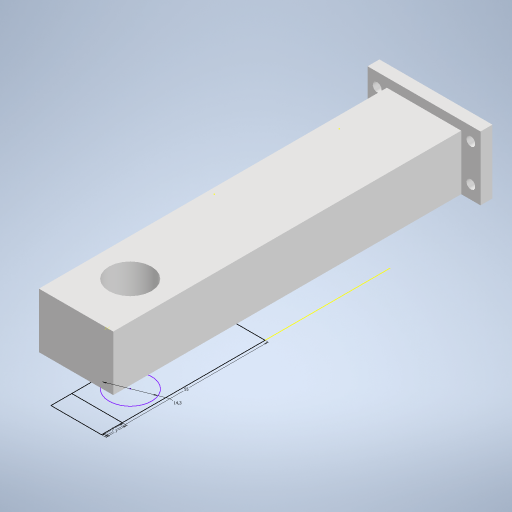
# Autodesk Inventor part: ramie_2
Saved by Autodesk Inventor 2023 (Build 270158000, 158)
## iProperties
Created: 2022-09-14
Part Number: ramie_2
Material: Generic
Document SubType Name: Modeling
Designer: Kamil
Density: 1 g/cm^3
Appearance: Default
Author: Kamil
Autodesk Inventor part; units mm, degrees
ref_plane "YZ Plane" through (0, 0, 0) normal (1, 0, 0) x (0, 1, 0)
ref_plane "XZ Plane" through (0, 0, 0) normal (0, 1, 0) x (-1, 0, 0)
ref_plane "XY Plane" through (0, 0, 0) normal (0, 0, 1) x (1, 0, 0)
sketch "Sketch14" plane through (0, 0, 0) normal (0, 0, 1) x (1, 0, 0)
  line L0 (0, 0) -> (17, 0)
  line L1 (17, 0) -> (17, 30)
  line L2 (17, 30) -> (0, 30)
  line L3 (0, 30) -> (0, 0)
  line L4 (-6, 36) -> (23, 36)
  line L5 (23, 36) -> (23, -6)
  line L6 (23, -6) -> (-6, -6)
  line L7 (-6, -6) -> (-6, 36)
  dimension "d55" = 17
  dimension "d56" = 30
  dimension "d57" = 6
  constraints: 16 end point, 4 parallel, 2 perpendicular, 1 horizontal, 3 other
  measures "d55" distance of L2.end L1.end
  measures "d56" distance of L1.end L0.end
  measures "d57" distance between parallel lines of L2 L4
extrude "Extrusion12" add sketch "Sketch14" against normal blind 3 contours L3 L2 L1 L0 | L4 L5 L6 L7
extrude "Extrusion13" add sketch "Sketch14" along normal blind 90 contours L3 L2 L1 L0
sketch "Sketch15" plane through (0, 0, 0) normal (0, -1, 0) x (1, 0, 0)
  line L0 (0, 0) -> (0, 90) projected
  line L1 (0, 90) -> (17.1111, 90)
  line L2 (0, 90) -> (17, 90)
  line L3 (17, 90) -> (17, 97)
  line L4 (17, 97) -> (0, 97)
  line L5 (0, 97) -> (0, 90)
  line L6 (17, 90) -> (0, 90) projected
  circle A0 centre (8.5, 78.8) radius 7.15
  line L7 (17, 0) -> (17, 90) projected
  line L8 (0, 97) -> (17, 97)
  line L9 (17, 97) -> (17, 42)
  line L10 (17, 42) -> (0, 42)
  line L11 (0, 42) -> (0, 97)
  dimension "d67" = 7
  dimension "d73" = 14.3
  dimension "d79" = 55
  constraints: 18 end point, 4 parallel, 3 horizontal, 2 perpendicular, 1 centre point, 1 point on line
  measures "d67" distance of L3.end L2.end
  measures "d73" diameter of A0
  measures "d79" distance of L8.end L9.end
extrude "Extrusion14" cut sketch "Sketch15" against normal blind 90 contours A0
extrude "Extrusion15" cut sketch "Sketch15" against normal blind 15.5 contours L0 L1 L7 L10
extrude "Extrusion17" add sketch "Sketch15" against normal blind 30 contours L5 L4 L3 L1
sketch "Sketch16" plane through (0, 0, 0) normal (0, -1, 0) x (1, 0, 0)
  line L0 (0, 0) -> (0, 97) projected
  line L1 (17, 0) -> (17, 97) projected
  line L2 (0, 97) -> (17, 97)
  line L3 (17, 97) -> (17, 90)
  line L4 (17, 90) -> (0, 90)
  line L5 (0, 90) -> (0, 97)
  dimension "d86" = 7
  constraints: 8 end point, 2 parallel, 1 horizontal, 1 perpendicular, 1 point on line
  measures "d86" distance of L2.end L3.end
extrude "Extrusion18" cut sketch "Sketch15" against normal blind 15.5 contours L5 L4 L3 L1
sketch "Sketch21" plane through (0, 15.5, 97) normal (0, 0, 1) x (1, 0, 0)
  line L0 (0, 14.5) -> (17, 14.5) projected
  line L1 (0, 14.5) -> (0, 16.5)
  line L2 (0, 16.5) -> (-2, 16.5)
  line L3 (17, 0) -> (19, 0)
  line L4 (19, 0) -> (19, -2)
  line L5 (-2, 16.5) -> (19, 16.5)
  line L6 (19, 16.5) -> (19, -2)
  line L7 (19, -2) -> (-2, -2)
  line L8 (-2, -2) -> (-2, 16.5)
  point P0 (0, -15.5)
  dimension "d109" = 2
  dimension "d110" = 2
  dimension "d111" = 2
  dimension "d112" = 2
  constraints: 16 end point, 3 perpendicular, 2 horizontal, 2 parallel, 1 vertical
  measures "d109" distance of L0.start L1.end
  measures "d110" distance of L1.end L2.end
  measures "d111" distance of L3.start L3.end
  measures "d112" distance of L3.end L4.end
extrude "Extrusion24" add sketch "Sketch21" against normal blind 97.9375
sketch "Sketch22" plane through (0, 0, 42) normal (0, 0, 1) x (1, 0, 0)
  line L0 (17, 13.5) -> (0, 13.5) projected
  line L1 (0, 13.5) -> (17.0001, 13.5)
  line L2 (17.0001, 13.5) -> (17.0001, 0)
  line L3 (17.0001, 0) -> (0, 0)
  line L4 (0, 0) -> (0, 13.5)
  constraints: 8 end point, 2 parallel, 1 horizontal, 1 perpendicular
extrude "Extrusion25" cut sketch "Sketch22" against normal blind 42
extrude "Extrusion26" cut sketch "Sketch15" against normal blind 97.9375 contours A0
sketch "Sketch23" plane through (0, 0, -3) normal (0, 0, -1) x (-1, 0, 0)
  line L0 (-28.2805, -15.4048) -> (9.4268, -15.4048)
  line L1 (9.4268, -15.4048) -> (9.4268, 47.594)
  line L2 (9.4268, 47.594) -> (-28.2805, 47.594)
  line L3 (-28.2805, 47.594) -> (-28.2805, -15.4048)
  point P0 (0, 0)
  constraints: 8 end point, 2 parallel, 1 horizontal, 1 perpendicular
extrude "Extrusion27" cut sketch "Sketch23" against normal blind 43
sketch "Sketch24" plane through (-2, 32, 97) normal (0, 1, 0) x (1, 0, 0)
  point P0 (2, 97)
sketch "Sketch25" plane through (-2, 32, 97) normal (0, 1, 0) x (1, 0, 0)
  point P0 (2, 97)
sketch "Sketch26" plane through (-2, 32, 97) normal (0, 1, 0) x (1, 0, 0)
  point P0 (2, 97)
sketch "Sketch27" plane through (-2, 32, 97) normal (0, 1, 0) x (1, 0, 0)
  point P0 (2, 97)
sketch "Sketch28" plane through (-2, 32, 97) normal (0, 1, 0) x (1, 0, 0)
  point P0 (2, 97)
sketch "Sketch29" plane through (-2, 32, 97) normal (0, 1, 0) x (1, 0, 0)
  point P0 (2, 97)
sketch "Sketch30" plane through (-2, 32, 97) normal (0, 1, 0) x (1, 0, 0)
  point P0 (2, 97)
  point P1 (21, 0)
  point P2 (0, 57)
sketch "Sketch31" plane through (0, 0, 40) normal (0, 0, -1) x (-1, 0, 0)
  line L0 (2, 13.5) -> (-19, 13.5) projected
  line L1 (-19, 32) -> (2, 32) projected
  line L2 (2, 13.5) -> (-19, 13.5)
  line L3 (-19, 13.5) -> (-19, 32)
  line L4 (-19, 32) -> (2, 32)
  line L5 (2, 32) -> (2, 13.5)
  point P0 (0, 0)
  point P1 (2, 32)
  constraints: 8 end point, 2 parallel, 1 horizontal, 1 perpendicular
extrude "Extrusion28" add sketch "Sketch31" along normal blind 43
sketch "Sketch33" plane through (-2, 13.5, 97) normal (0, 0, 1) x (1, 0, 0)
  line L0 (0, 0) -> (21, 0) projected
  line L1 (0, 0) -> (-2, 0)
  line L2 (-2, 0) -> (-2, 18.5)
  line L3 (-2, 18.5) -> (0, 18.5)
  line L4 (0, 18.5) -> (0, 0)
  line L5 (21, 0) -> (21, 18.5) projected
  line L6 (21, 0) -> (23, 0)
  line L7 (23, 0) -> (23, 18.5)
  line L8 (23, 18.5) -> (21, 18.5)
  line L9 (21, 18.5) -> (21, 0)
  point P0 (2, -13.5)
  dimension "d123" = 2
  dimension "d124" = 2
  constraints: 16 end point, 4 parallel, 2 horizontal, 2 perpendicular
  measures "d123" distance of L2.end L3.end
  measures "d124" distance of L8.end L7.end
extrude "Extrusion29" add sketch "Sketch33" against normal blind 100
sketch "Sketch37" plane through (0, 0, -3) normal (0, 0, -1) x (-1, 0, 0)
  line L0 (-21, 32) -> (-21, 13.5) projected
  line L1 (4, 13.5) -> (-21, 13.5) projected
  line L2 (-21, 32) -> (4, 32)
  line L3 (4, 32) -> (4, 13.5)
  line L4 (4, 13.5) -> (-21, 13.5)
  line L5 (-21, 13.5) -> (-21, 32)
  point P0 (0, 0)
  constraints: 8 end point, 2 parallel, 1 horizontal, 1 perpendicular
extrude "Extrusion30" add sketch "Sketch37" along normal blind 17
sketch "Sketch38" plane through (0, 0, -20) normal (0, 0, -1) x (-1, 0, 0)
  line L0 (4, 13.5) -> (-21, 13.5) projected
  line L1 (4, 13.5) -> (10.5, 13.5)
  line L2 (10.5, 13.5) -> (10.5, 32)
  line L3 (10.5, 32) -> (4, 32)
  line L4 (4, 32) -> (4, 13.5)
  line L5 (-21, 13.5) -> (-21, 32) projected
  line L6 (-21, 13.5) -> (-27.5, 13.5)
  line L7 (-27.5, 13.5) -> (-27.5, 32)
  line L8 (-27.5, 32) -> (-21, 32)
  line L9 (-21, 32) -> (-21, 13.5)
  line L10 (-27.5, 32) -> (10.5, 32)
  line L11 (10.5, 32) -> (10.5, 36)
  line L12 (10.5, 36) -> (-27.5, 36)
  line L13 (-27.5, 36) -> (-27.5, 32)
  line L14 (-24.25, 13.5) -> (-24.25, 18)
  line L15 (-24.25, 36) -> (-24.25, 30.5)
  line L16 (7.25, 36) -> (7.25, 30.5)
  line L17 (7.25, 13.5) -> (7.25, 18)
  circle A0 centre (-24.25, 30.5) radius 1.5
  circle A1 centre (-24.25, 18) radius 1.5
  circle A2 centre (7.25, 18) radius 1.5
  circle A3 centre (7.25, 30.5) radius 1.5
  line L18 (-24.25, 31.5) -> (-24.25, 30.5)
  line L19 (7.25, 31.5) -> (7.25, 30.5)
  line L20 (-27.5, 36) -> (10.5, 36)
  line L21 (10.5, 36) -> (10.5, 35)
  line L22 (10.5, 35) -> (-27.5, 35)
  line L23 (-27.5, 35) -> (-27.5, 36)
  line L24 (7.25, 35) -> (10.5, 35)
  line L25 (10.5, 35) -> (10.5, 32)
  line L26 (10.5, 32) -> (7.25, 32)
  line L27 (7.25, 32) -> (7.25, 35)
  point P0 (0, 0)
  point P1 (7.25, 32)
  point P2 (7.25, 32)
  point P3 (7.25, 32)
  point P4 (7.25, 35)
  dimension "d132" = 4.5
  dimension "d135" = 4.5
  dimension "d137" = 3
  dimension "d138" = 3
  dimension "d142" = 1
  dimension "d143" = 1
  constraints: 52 end point, 10 parallel, 7 point on line, 6 perpendicular, 5 horizontal, 5 vertical, 4 centre point, 4 coincident, 2 midpoint
  measures "d132" distance of L14.start L14.end
  measures "d135" distance of L17.start L17.end
  measures "d137" diameter of A1
  measures "d138" diameter of A2
  measures "d142" distance of L18.start L18.end
  measures "d143" distance of L19.start L19.end
extrude "Extrusion31" add sketch "Sketch38" along normal blind 4 contours L4 L3 L2 L1 | L0 L5 L10 L4 | L6 L7 L8 L5 | L10 L8 L15 L22 L16 L3 | L16 L22 L11 L3 | L8 L13 L22 L15
body "Solid2"
